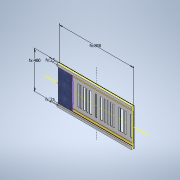
# Autodesk Inventor part: ferrite_layer_dex_0R2
Saved by Autodesk Inventor 2021 (Build 250183000, 183)
## iProperties
Created: 2021-01-27
Part Number: ferrite_layer_dex_0R2
Material: Generic
Document SubType Name: Modeling
Designer: pduy110
Density: 1 g/cm^3
Appearance: Default
Author: pduy110
Autodesk Inventor part; units mm, degrees
ref_plane "YZ Plane" through (0, 0, 0) normal (1, 0, 0) x (0, 1, 0)
ref_plane "XZ Plane" through (0, 0, 0) normal (0, 1, 0) x (-1, 0, 0)
ref_plane "XY Plane" through (0, 0, 0) normal (0, 0, 1) x (1, 0, 0)
sketch "ferrite_layer_outline_sketch" plane through (0, 0, 0) normal (0, 0, 1) x (1, 0, 0)
  line L0 (0, 200) -> (800, 200)
  line L1 (800, 200) -> (800, -200)
  line L2 (800, -200) -> (0, -200)
  line L3 (0, -200) -> (0, 200)
  line L4 (-160, 0) -> (960, 0) projected
  line L5 (400, 200) -> (400, -200) construction
  line L6 (400, 366.8869) -> (400, -324.3455) construction
  line L7 (400, 200) -> (400, -200)
  point P0 (0, 0)
  point P1 (0, 0)
  point P2 (0, 0)
  point P3 (0, 0)
  point P4 (20, 0)
  dimension "d0" = 800
  dimension "d1" = 400
  constraints: 14 end point, 3 coincident, 3 midpoint, 3 point on line, 2 parallel, 1 collinear, 1 horizontal, 1 perpendicular
  measures "d0" distance between parallel lines of L1 L3
  measures "d1" distance between parallel lines of L2 L0
extrude "Extrusion8" add sketch "ferrite_layer_outline_sketch" along normal blind 4
ref_plane "acrylic_sheet_plane" through (0, 0, 4) normal (0, 0, 1) x (1, 0, 0)
sketch "Sketch4" plane through (0, 0, 4) normal (0, 0, 1) x (1, 0, 0)
  line L0 (14.5, 109) -> (29.5, 109)
  line L1 (29.5, 109) -> (29.5, -109)
  line L2 (29.5, -109) -> (14.5, -109)
  line L3 (14.5, -109) -> (14.5, 109)
  line L4 (-12.6534, 0) -> (47.471, 0)
  line L5 (0, 200) -> (0, -200) projected
  line L6 (800, 200) -> (0, 200) projected
  line L7 (0, -200) -> (800, -200) projected
  point P0 (0, 0)
  point P1 (14.5, 0)
  point P2 (0, 0)
  dimension "d43" = 15
  dimension "d44" = 218
  dimension "d45" = 14.5
  constraints: 10 end point, 2 horizontal, 2 midpoint, 2 parallel, 2 point on line, 1 perpendicular
  measures "d43" distance between parallel lines of L1 L3
  measures "d44" distance between parallel lines of L2 L0
  measures "d45" distance between parallel lines of L5 L3
extrude "Extrusion9" cut sketch "Sketch4" against normal through all
pattern_linear "Rectangular Pattern 7 fer" count 7 spacing 126 along (1, 0, 0) of "Extrusion9"
pattern_linear "Rectangular Pattern 8 fer" count 8 spacing 108 along (1, 0, 0) of "Extrusion9"
pattern_linear "pattern_test_#_of_ferrites 9 fer" count 9 spacing 94.5 along (1, 0, 0) of "Extrusion9"
pattern_linear "Rectangular Pattern 10 fer" [suppressed]
pattern_linear "Rectangular Pattern 13" count 13 spacing 63 along (1, 0, 0) of "Extrusion9"
sketch "Sketch5" plane through (0, 0, 4) normal (0, 0, 1) x (1, 0, 0)
  line L0 (0, 200) -> (0, -200) projected
  line L1 (0, 150) -> (800, 150)
  line L2 (800, -200) -> (800, 200) projected
  line L3 (800, 200) -> (0, 200) projected
  line L4 (0, -200) -> (800, -200) projected
  line L5 (0, -150) -> (800, -150)
  point P0 (0, 0)
  dimension "d66" = 50
  dimension "d68" = 50
  constraints: 4 end point, 4 point on line, 1 horizontal, 1 perpendicular
  measures "d66" distance between parallel lines of L3 L1
  measures "d68" distance between parallel lines of L4 L5
extrude "Extrusion10" add sketch "Sketch5" along normal blind 4.5 contours L3 L2 L1 L0 | L5 L2 L4 L0
ref_plane "lower test Plane" through (0, 0, 8.5) normal (0, 0, 1) x (1, 0, 0)
sketch "Sketch7" plane through (0, 0, 8.5) normal (0, 0, 1) x (1, 0, 0)
  line L0 (0, 200) -> (0, -200) projected
  line L1 (0, 175) -> (800, 175)
  line L2 (800, -200) -> (800, 200) projected
  line L3 (0, -175) -> (800, -175)
  line L4 (800, 200) -> (0, 200) projected
  line L5 (0, -200) -> (800, -200) projected
  line L6 (148.5652, 175) -> (148.5652, -175)
  point P0 (0, 0)
  dimension "d77" = 25
  dimension "d78" = 25
  constraints: 6 end point, 4 point on line, 2 horizontal, 1 perpendicular
  measures "d77" distance between parallel lines of L1 L4
  measures "d78" distance between parallel lines of L5 L3
extrude "wall extrusion" add sketch "Sketch7" along normal blind 15 contours L4 L2 L1 L0 | L3 L2 L5 L0
extrude "Extrusion14" add sketch "Sketch7" along normal blind 3 contours L1 L6 L3 L0
equation "\"d0\" = track_length"
equation "\"d1\" = track_width"
equation "\"d43\" = ferrite_width"
equation "\"d44\" = ferrite_length"
equation "\"d45\" = gap_distance"
equation "\"d50\" = parameter_5"
equation "\"d62\" = test_parameter_5"
equation "\"track_length\" = 800"
equation "\"track_width\" = 400"
equation "\"gap_distance\" = 14.5"
equation "\"ferrite_length\" = 218"
equation "\"ferrite_width\" = 15"
equation "\"ferrite_height\" = 8"
equation "\"acrylic_sheet_8mm\" = 8"
equation "\"parameter_5\" = 126"
equation "\"test_parameter_5\" = 94.5"
body "Solid8"
